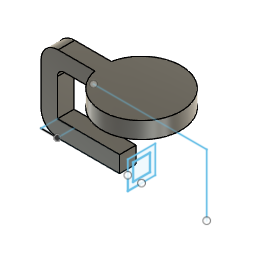
RadioGlobe-NS-Encoder-Clamp v25 (Autodesk Fusion 360 design; units mm, degrees)
Autodesk Fusion 360 part; units mm, degrees
sketch "Sketch1" plane through (0, 0, 0) normal (0, 0, 1) x (1, 0, 0)
  circle A0 centre (0, 0) radius 14.8
  circle A1 centre (0, 0) radius 12
  line L0 (0, 0) -> (14.8, 0) construction
  circle A2 centre (0, 0) radius 18
  line L1 (0, 0) -> (75, 0) construction
  line L2 (0, 0) -> (26.9258, 0) construction
  line L3 (0, 0) -> (25, 0) construction
  line L4 (0, 0) -> (22.2384, 0) construction
  line L5 (0, 0) -> (26.6458, 0) construction
  line L6 (0, 0) -> (55, 0) construction
  line L7 (-6, 10.3923) -> (-7.4, 12.8172)
  line L8 (0, 0) -> (31.8904, 0) construction
  line L9 (0, 0) -> (8.4889, -12.1235)
  dimension "d2" = 29.6
  dimension "d3" = 24
  dimension "d25" = 36
  dimension "d43" = 120
  dimension "d46" = 55
  constraint concentric A0 A1
  constraint horizontal L0
  constraint coincident A0.centre A1.centre
  constraint horizontal L1
  constraint horizontal L2
  constraint horizontal L3
  constraint horizontal L4
  constraint horizontal L5
  constraint horizontal L6
  constraint coincident A1 L7.start
  constraint coincident A0 L7.end
  constraint horizontal L8
  constraint coincident A0 L9.end
  measures "d2" diameter of A0
  measures "d3" diameter of A1
  measures "d25" diameter of A2
  measures "d43" angle of L5 L7
  measures "d46" angle of L8 L9
sketch "Sketch6" plane through (0, 0, 0) normal (1, 0, 0) x (0, 1, 0)
  circle A0 centre (0, -102) radius 100
  dimension "d41" = 200
  measures "d41" diameter of A0
extrude "Extrude1" add sketch "Sketch1" along normal blind 11 contours A0 A1 L7 L9 | A0 A1 L7 L9 makes body 1
extrude "Extrude2" add sketch "Sketch1" along normal blind 8 separate body makes body 2
extrude "Extrude3" add sketch "Sketch1" along normal blind 2 contours A1 bodies 1
sketch "Sketch2" plane through (0, 0, 2) normal (0, 0, 1) x (-1, 0, 0)
  circle A0 centre (0, 0) radius 12
  circle A1 centre (0, 0) radius 4
  constraint coincident A0.centre A1.centre
extrude "Extrude4" add sketch "Sketch2" along normal blind 8.75 contours A1 bodies 1
sketch "Sketch3" plane through (0, 0, 10.75) normal (0, 0, 1) x (-1, 0, 0)
  circle A0 centre (0, 0) radius 4
  circle A1 centre (0, 0) radius 2.1
  dimension "d12" = 4.2
  constraint coincident A0.centre A1.centre
  measures "d12" diameter of A1
extrude "Extrude5" cut sketch "Sketch3" against normal blind 2 contours A1 bodies 1
extrude "Extrude7" add sketch "Sketch1" along normal blind 12.5 and the other way blind 0 contours A0 A1 L7 L9 picked at (-6.269, 12.3288) bodies 1 2
sketch "Sketch5" plane through (0, 0, 0) normal (0, 1, 0) x (1, 0, 0)
  line L0 (0, -7) -> (4.5, -7)
  line L1 (0, -7) -> (-4.5, -7)
  line L2 (-4.5, -7) -> (-4.5, 0)
  line L3 (-4.5, 0) -> (4.5, 0)
  line L4 (4.5, 0) -> (4.5, -7)
  line L5 (-3, -1.5) -> (3, -1.5)
  line L6 (3, -1.5) -> (3, -5.5)
  line L7 (0, -5.5) -> (3, -5.5)
  line L8 (0, -5.5) -> (-3, -5.5)
  line L9 (-3, -5.5) -> (-3, -1.5)
  line L10 (0, 0) -> (0, 102)
  line L11 (0, 102) -> (50, 102)
  line L12 (-2.9, -1.6) -> (2.9, -1.6)
  line L13 (2.9, -1.6) -> (2.9, -5.4)
  line L14 (0, -5.4) -> (2.9, -5.4)
  line L15 (0, -5.4) -> (-2.9, -5.4)
  line L16 (-2.9, -5.4) -> (-2.9, -1.6)
  dimension "d26" = 7
  dimension "d27" = 4.5
  dimension "d28" = 4.5
  dimension "d29" = 7
  dimension "d30" = 1.5
  dimension "d31" = 102
  dimension "d34" = 1.6
  constraint perpendicular L0 L2
  constraint perpendicular L0 L4
  constraint coincident L10.start origin
  constraint perpendicular L3 L10
  constraint perpendicular L10 L11
  measures "d26" distance of L10.start L0.start
  measures "d27" distance of L0.start L0.end
  measures "d28" distance of L0.start L1.end
  measures "d29" distance of L1.end L2.end
  measures "d31" distance of L10.start L10.end
revolve "Revolve1" add sketch "Sketch5" angle 15 about axis through (0, 0, -102) along (1, 0, 0) second angle -7 contours L0 L1 L2 L3 L4 bodies 1
revolve "Revolve2" add sketch "Sketch5" angle 10 about axis through (0, 0, -102) along (1, 0, 0) second angle -85 separate body contours L12 L13 L14 L15 L16 makes body 3
sketch "Sketch7" plane through (0, 0, 0) normal (1, 0, 0) x (0, 1, 0)
sketch "Sketch8" plane through (0, 0, 0) normal (1, 0, 0) x (0, 1, 0)
  line L0 (-4, 4) -> (-4, 0)
  line L1 (-4, 0) -> (0, 0)
  line L2 (-4, 0) -> (4, 0)
  line L3 (4, 0) -> (4, 8)
  line L4 (4, 8) -> (-4, 8)
  line L5 (-4, 8) -> (-4, 0)
  line L6 (-2.5, 1.5) -> (2.5, 1.5)
  line L7 (2.5, 1.5) -> (2.5, 6.5)
  line L8 (2.5, 6.5) -> (-2.5, 6.5)
  line L9 (-2.5, 6.5) -> (-2.5, 1.5)
  line L10 (-2.4, 1.6) -> (2.4, 1.6)
  line L11 (2.4, 1.6) -> (2.4, 6.4)
  line L12 (2.4, 6.4) -> (-2.4, 6.4)
  line L13 (-2.4, 6.4) -> (-2.4, 1.6)
  dimension "d48" = 8
  dimension "d49" = 8
  dimension "d50" = -1.5
  dimension "d62" = -1.6
  constraint vertical L0
  constraint horizontal L1
  constraint horizontal L2
  constraint vertical L3
  constraint horizontal L4
  constraint vertical L5
  measures "d48" distance of L0.end L2.end
  measures "d49" distance of L0.end L4.end
extrude "Extrude8" add sketch "Sketch8" along normal blind -7 and the other way blind 22 contours L0 L1 L2 L3 L4 L5 bodies 1
extrude "Extrude11" add sketch "Sketch8" along normal blind -4 and the other way blind 26.9 separate body contours L10 L11 L12 L13 makes body 4
sketch "Sketch10" plane through (0, 0, 1.6) normal (0, 0, -1) x (1, 0, 0)
  line L0 (-4, -2.4) -> (-4, 2.4)
  line L1 (-4, 2.4) -> (-26.9, 2.4)
  line L2 (-26.9, 2.4) -> (-26.9, -2.4)
  line L3 (-26.9, -2.4) -> (-4, -2.4)
  line L4 (-22.1, 2.4) -> (-26.9, 2.4)
  line L5 (-26.9, 2.4) -> (-26.9, -2.4)
  line L6 (-26.9, -2.4) -> (-22.1, -2.4)
  line L7 (-22.1, -2.4) -> (-22.1, 2.4)
  dimension "d69" = 4.8
  dimension "d70" = 4.8
  constraint horizontal L4
  constraint vertical L5
  constraint horizontal L6
  constraint vertical L7
  constraint coincident L1 L4.start
  measures "d69" distance of L4.start L1.end
  measures "d70" distance of L4.start L6.end
sketch "Sketch12" plane through (0, 0, 6.4) normal (0, 0, -1) x (1, 0, 0)
  line L0 (-22.1, -2.4) -> (-22.1, 2.4)
  line L1 (-22.1, 2.4) -> (-26.9, 2.4)
  line L2 (-26.9, 2.4) -> (-26.9, -2.4)
  line L3 (-26.9, -2.4) -> (-22.1, -2.4)
  line L4 (-26.9, 2.4) -> (-22.1, 2.4)
  line L5 (-22.1, -2.4) -> (-26.9, -2.4)
  line L6 (-26.9, -2.4) -> (-26.9, 2.4)
  line L7 (-11.2468, -2.4) -> (-22.1, -2.4)
  line L8 (-22.1, -2.4) -> (-22.1, 2.4)
  circle A0 centre (0, 0) radius 10
  arc A1 (-11.2468, -2.4) -> (-11.2468, 2.4) centre (0, 0) ccw
  line L9 (-22.1, 2.4) -> (-11.2468, 2.4)
  line L10 (-4, 2.4) -> (-4, -2.4)
  line L11 (-4, -2.4) -> (-26.9, -2.4)
  line L12 (-26.9, -2.4) -> (-26.9, 2.4)
  line L13 (-26.9, 2.4) -> (-4, 2.4)
  dimension "d82" = 20
  dimension "d83" = 23
  constraint horizontal L4
  constraint horizontal L5
  constraint vertical L6
  constraint coincident L0.start L3.end
  constraint coincident L1.end L2.start
  constraint horizontal L9
  constraint horizontal L7
  constraint vertical L8
  constraint coincident L0.end L1.start
  constraint coincident A0.centre A1.centre
  measures "d82" diameter of A0
  measures "d83" diameter of A1
extrude "Extrude16" add sketch "Sketch12" along normal blind -17.5 and the other way blind 12.7 separate body contours L0 L1 L2 L3 L4 L5 L6 L8 L11 L12 L13 | L0 L7 L8 A0 L9 L11 L13 | A0 A1 L11 L13 makes body 5
extrude "Extrude15" add sketch "Sketch12" along normal blind -12.7 and the other way blind 0 contours L0 L1 L2 L3 L4 L5 L6 L8 L11 L12 L13 bodies 4 5
extrude "Extrude17" add sketch "Sketch12" along normal blind -13.7 and the other way blind 17.5 contours A0 L10 L11 L13 | A0 L10 L11 L13 bodies 4
sketch "Sketch13" plane through (0, 0, 0) normal (0, 1, 0) x (1, 0, 0)
  line L0 (19, 0) -> (19, -18)
  line L1 (19, -18) -> (-14, -18)
  constraint vertical L0
  constraint perpendicular L0 L1
extrude "Extrude18" cut sketch "Sketch8" along normal blind -33 and the other way blind 4 contours L6 L7 L8 L9 | L10 L11 L12 L13 bodies 1
fillet "Fillet7" radius 5 2 edges at (-26.9, 0, 1.6) (-26.9, 0, 23.9) on bodies 4
fillet "Fillet10" radius 2 1 edges at (-22.1, 0, 19.1) on bodies 4
sketch "Sketch15" plane through (0, 0, 6.4) normal (0, 0, -1) x (1, 0, 0)
  line L0 (-0.0359, 8.0622) -> (-7.5359, 21.0526)
  line L1 (-7.5359, 21.0526) -> (-14.4641, 17.0526)
  line L2 (-14.4641, 17.0526) -> (-6.9641, 4.0622)
  line L3 (-6.9641, 4.0622) -> (-0.0359, 8.0622)
sketch "Sketch16" plane through (0, 0, 6.4) normal (0, 0, -1) x (1, 0, 0)
extrude "Extrude19" add sketch "Sketch15" along normal blind 6.4 and the other way blind 1.6 separate body makes body 6
sketch "Sketch17" plane through (-11, -19.0526, 0) normal (-0.5, -0.866025, 0) x (0.866025, -0.5, 0)
  line L0 (-4, 8) -> (-4, 0)
  line L1 (-4, 0) -> (4, 0)
  line L2 (4, 0) -> (4, 8)
  line L3 (4, 8) -> (-4, 8)
  line L4 (-2.5, 1.5) -> (2.5, 1.5)
  line L5 (2.5, 1.5) -> (2.5, 6.5)
  line L6 (2.5, 6.5) -> (-2.5, 6.5)
  line L7 (-2.5, 6.5) -> (-2.5, 1.5)
  dimension "d124" = -1.5
extrude "Extrude20" cut sketch "Sketch17" against normal blind 18 contours L4 L5 L6 L7 bodies 1 6
hidden bodies 1 3 6
